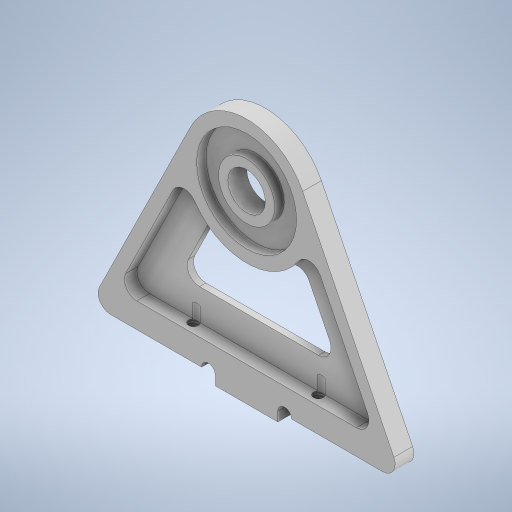
# Autodesk Inventor part: kosipitch
Saved by Autodesk Inventor 2024 (Build 280153000, 153)
## iProperties
Created: 2024-07-10
Part Number: kosipitch
Material: 一般
Document SubType Name: Modeling
Designer: right
Density: 1 g/cm^3
Appearance: 既定
Author: right
Autodesk Inventor part; units mm, degrees
ref_plane "YZ Plane" through (0, 0, 0) normal (1, 0, 0) x (0, 1, 0)
ref_plane "XZ Plane" through (0, 0, 0) normal (0, 1, 0) x (-1, 0, 0)
ref_plane "XY Plane" through (0, 0, 0) normal (0, 0, 1) x (1, 0, 0)
sketch "スケッチ1" plane through (0, 0, 0) normal (0, 0, 1) x (1, 0, 0)
  circle A0 centre (0, 0) radius 3
  circle A1 centre (0, 0) radius 10
  line L0 (-25, -28) -> (25, -28)
  line L1 (-5, -28) -> (5, -28)
  line L2 (5, -28) -> (5, -29.5)
  line L3 (5, -29.5) -> (-5, -29.5)
  line L4 (-5, -29.5) -> (-5, -28)
  circle A2 centre (-6.1, -28) radius 1.1
  circle A3 centre (6.1, -28) radius 1.1
  line L5 (-25, -28) -> (-8.9641, 4.4322)
  line L6 (8.9641, 4.4322) -> (25, -28)
  line L7 (0, 0) -> (0, -28) construction
  point P0 (0, -29.5)
  point P1 (-7.2, -28)
  point P2 (7.2, -28)
  dimension "d5" = 2.2
  dimension "d6" = 2.2
  dimension "d0" = 6
  dimension "d1" = 20
  dimension "d2" = 28
  dimension "d3" = 1.5
  dimension "d4" = 10
  dimension "d7" = 50
  constraints: 16 end point, 3 point on line, 2 centre point, 2 coincident, 2 horizontal, 2 midpoint, 2 parallel, 2 point on circle, 2 tangent, 1 perpendicular, 1 vertical alignment, 7 other
  measures "d0" diameter of A0
  measures "d1" diameter of A1
  measures "d2" distance from line of A0.centre L0
  measures "d3" distance between parallel lines of L0 L3
  measures "d4" distance of L2.end L3.end
  measures "d7" distance of L0.start L0.end
extrude "押し出し1" add sketch "スケッチ1" along normal blind 3 contours A1 | A1 L6 L0 A3 A2 L5 | L2 L3 L4 L0
fillet "フィレット1" radius 2 2 edges at (25, -28, 1.5) (-25, -28, 1.5)
sketch "スケッチ2" plane through (-7.2, -28, 0) normal (0, -1, 0) x (1, 0, 0)
  line L0 (2.2, 0) -> (2.2, 3) projected
  line L1 (12.2, 0) -> (12.2, 3) projected
  point P0 (7.2, 0)
  point P1 (-2.8, 1.5)
  point P2 (17.2, 1.5)
  point P3 (2.2, 1.5)
  point P4 (12.2, 1.5)
  dimension "d11" = 5
  dimension "d12" = 5
  constraints: 2 horizontal alignment, 2 midpoint
  measures "d11" distance from line of L1 point (17.2, 1.5)
  measures "d12" distance from line of point (-2.8, 1.5) L0
hole "穴1" at (-10, -28, 1.5) at (10, -28, 1.5) direction (0, 1, 0) diameter 1.567 depth 6.3 tip angle 118 thread size "M2x0.4" class "6H" standard "ISO Metric profile"
sketch "スケッチ3" plane through (0, 0, 3) normal (0, 0, 1) x (1, 0, 0)
  arc A0 (-23.5728, -25.1136) -> (-21.78, -28) centre (-21.78, -26) ccw projected
  line L0 (-21.78, -28) -> (-7.2, -28) projected
  arc A1 (-5, -28) -> (-7.2, -28) centre (-6.1, -28) ccw projected
  line L1 (-5, -28) -> (-5, -29.5) projected
  line L2 (-5, -29.5) -> (5, -29.5) projected
  line L3 (5, -29.5) -> (5, -28) projected
  arc A2 (7.2, -28) -> (5, -28) centre (6.1, -28) ccw projected
  line L4 (7.2, -28) -> (21.78, -28) projected
  arc A3 (21.78, -28) -> (23.5728, -25.1136) centre (21.78, -26) ccw projected
  line L5 (23.5728, -25.1136) -> (8.9641, 4.4322) projected
  arc A4 (8.9641, 4.4322) -> (-8.9641, 4.4322) centre (0, 0) ccw projected
  line L6 (-8.9641, 4.4322) -> (-23.5728, -25.1136) projected
  circle A5 centre (0, 0) radius 3 projected
  line L7 (-17.5711, -24) -> (17.5711, -24)
  line L8 (19.3639, -21.1136) -> (9.8306, -1.8327)
  line L9 (-19.3639, -21.1136) -> (-9.8306, -1.8327)
  circle A6 centre (0, 0) radius 10
  line L10 (23.5728, -25.1136) -> (8.9641, 4.4322) projected
  arc A7 (-19.3639, -21.1136) -> (-17.5711, -24) centre (-17.5711, -22) ccw
  arc A8 (17.5711, -24) -> (19.3639, -21.1136) centre (17.5711, -22) ccw
  line L11 (-5.3486, -4.0488) -> (-12.7411, -19)
  line L12 (-12.7411, -19) -> (12.7411, -19)
  line L13 (12.7411, -19) -> (5.3486, -4.0488)
  point P0 (6.9173, -7.2215)
  point P1 (-6.9173, -7.2215)
  dimension "d20" = 2
  dimension "d21" = 2
  dimension "d22" = 4
  dimension "d23" = 2
  dimension "d27" = 20
  dimension "d33" = 5
  constraints: 12 end point, 6 point on circle, 4 tangent, 3 centre point, 1 coincident, 1 equal radius, 1 horizontal, 1 parallel, 2 other
  measures "d20" distance between parallel lines of L6 L9
  measures "d21" distance between parallel lines of L5 L8
  measures "d22" distance between parallel lines of L0 L7
  measures "d23" radius of A7
  measures "d27" diameter of A6
  measures "d33" distance between parallel lines of L9 L11
extrude "押し出し2" cut sketch "スケッチ3" against normal blind 2 contours A6 L11 L12 L13 L8 A8 L7 A7 L9 | A6 L13 L12 L11
fillet "フィレット2" radius 2 2 edges at (-9.8306, -1.8327, 2) (9.8306, -1.8327, 2)
sketch "スケッチ4" plane through (0, 0, 3) normal (0, 0, 1) x (1, 0, 0)
  circle A0 centre (0, 0) radius 10
  arc A1 (-8.3205, -5.547) -> (8.3205, -5.547) centre (0, 0) ccw projected
  circle A2 centre (0, 0) radius 8
  circle A3 centre (0, 0) radius 3 projected
  circle A4 centre (0, 0) radius 4.5
  dimension "d28" = 2
  dimension "d30" = 1.5
  constraints: 3 centre point, 1 coincident, 1 concentric
  measures "d28" radial gap between concentric circles of A0 A2
  measures "d30" radial gap between concentric circles of A3 A4
extrude "押し出し3" cut sketch "スケッチ4" against normal blind 1.5 contours A2
extrude "押し出し4" cut sketch "スケッチ3" against normal through all contours A6 L13 L12 L11
fillet "フィレット3" radius 2 4 edges at (-6.9173, -7.2215, 0.5) (6.9173, -7.2215, 0.5) (-12.7411, -19, 0.5) (12.7411, -19, 0.5)
equation "\"d12\" = d11"
